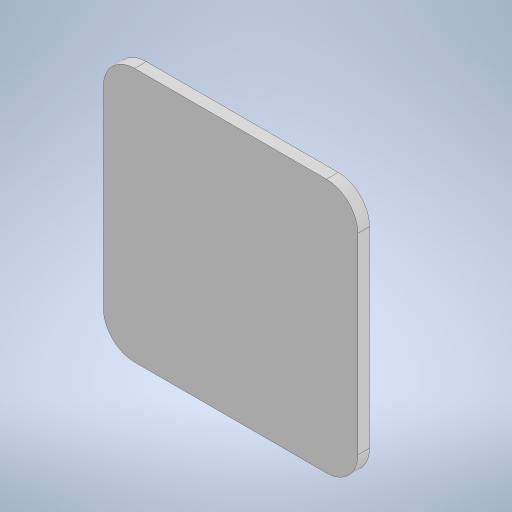
# Autodesk Inventor part: square_with_fillet_65mm
Saved by Autodesk Inventor 2024 (Build 280153000, 153)
## iProperties
Created: 2024-01-31
Part Number: square_with_fillet_65mm
Material: Generic
Document SubType Name: Modeling
Designer: Pintu
Density: 1 g/cm^3
Appearance: Default
Author: Pintu
Autodesk Inventor part; units mm, degrees
ref_plane "YZ Plane" through (0, 0, 0) normal (1, 0, 0) x (0, 1, 0)
ref_plane "XZ Plane" through (0, 0, 0) normal (0, 1, 0) x (-1, 0, 0)
ref_plane "XY Plane" through (0, 0, 0) normal (0, 0, 1) x (1, 0, 0)
sketch "Sketch1" plane through (0, 0, 0) normal (0, 0, 1) x (1, 0, 0)
  line L0 (-32.5, 32.5) -> (32.5, 32.5)
  line L1 (32.5, 32.5) -> (32.5, -32.5)
  line L2 (32.5, -32.5) -> (-32.5, -32.5)
  line L3 (-32.5, -32.5) -> (-32.5, 32.5)
  line L4 (-32.5, 32.5) -> (32.5, -32.5) construction
  line L5 (32.5, 32.5) -> (-32.5, -32.5) construction
  point P0 (0, 0)
  dimension "d0" = 65
  dimension "d1" = 65
  constraints: 12 end point, 2 midpoint, 2 parallel, 1 horizontal, 1 perpendicular
  measures "d0" distance of L1.end L2.end
  measures "d1" distance of L0.end L1.end
extrude "Extrusion1" add sketch "Sketch1" along normal blind 3
fillet "Fillet1" radius 8 4 edges at (-32.5, -32.5, 1.5) (32.5, -32.5, 1.5) (32.5, 32.5, 1.5) (-32.5, 32.5, 1.5)
sketch "Sketch2" plane through (0, 0, 0) normal (0, 0, -1) x (-1, 0, 0)
  circle A0 centre (0, 0) radius 15
  dimension "d5" = 30
  constraints: 1 centre point, 1 coincident
  measures "d5" diameter of A0
extrude "Extrusion2" add sketch "Sketch2" along normal blind 10
fillet "Fillet2" radius 3 1 edges at (15, 0, 0)
fillet "Fillet3" radius 1.5 1 edges at (15, 0, -10)
body "Solid1"
